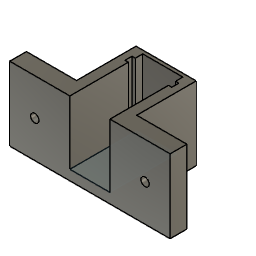
clock_light_holder (Autodesk Fusion 360 design; units mm, degrees)
Autodesk Fusion 360 part; units mm, degrees
sketch "Skizze1" plane through (0, 0, 0) normal (0, 0, 1) x (1, 0, 0)
  line L0 (0, 24) -> (16, 24)
  line L1 (16, 0) -> (0, 0)
  line L2 (2, 22) -> (14, 22)
  line L3 (0, 24) -> (-1, 24)
  line L4 (-1, 24) -> (-1, 0)
  line L5 (-1, 0) -> (0, 0)
  line L6 (16, 24) -> (17, 24)
  line L7 (17, 24) -> (17, 0)
  line L8 (17, 0) -> (16, 0)
  line L9 (2, 22) -> (1, 22)
  line L10 (1, 22) -> (1, 20)
  line L11 (1, 20) -> (2, 20)
  line L12 (15, 20) -> (15, 22)
  line L13 (15, 22) -> (14, 22)
  line L14 (15, 20) -> (2, 20)
  line L15 (2, 20) -> (2, 0)
  line L16 (14, 20) -> (14, 0)
  constraint coincident L1.end L5.end
  constraint perpendicular L3 L4
  constraint perpendicular L6 L7
  constraint perpendicular L9 L10
  constraint perpendicular L11 L12
  constraint coincident L1 L15.end
  constraint perpendicular L1 L15
  constraint coincident L14 L16.start
  constraint coincident L1 L16.end
  constraint perpendicular L1 L16
extrude "Extrusion1" add sketch "Skizze1" along normal blind 2
sketch "Skizze2" plane through (0, 0, 2) normal (0, 0, 1) x (-1, 0, 0)
  line L0 (-17, -24) -> (1, -24)
  line L1 (1, -24) -> (1, 0)
  line L2 (1, 0) -> (-17, 0)
  line L3 (-17, 0) -> (-17, -24)
  line L4 (-2, 0) -> (-2, -20)
  line L5 (-2, -20) -> (-1, -20)
  line L6 (-1, -20) -> (-1, -22)
  line L7 (-1, -22) -> (-15, -22)
  line L8 (-15, -22) -> (-15, -20)
  line L9 (-15, -20) -> (-14, -20)
  line L10 (-14, -20) -> (-14, 0)
  line L11 (-2, -20) -> (-14, -20)
  constraint coincident L2 L4.start
  constraint perpendicular L0 L4
  constraint perpendicular L4 L5
  constraint perpendicular L5 L6
  constraint perpendicular L6 L7
  constraint perpendicular L7 L8
  constraint perpendicular L8 L9
  constraint coincident L2 L10.end
  constraint perpendicular L2 L10
  constraint perpendicular L10 L11
extrude "Extrusion2" add sketch "Skizze2" along normal blind 1 contours L0 L1 L2 L3 L4 L5 L6 L7 L8 L9 L10 | L2 L4 L10 L11
sketch "Skizze3" plane through (0, 0, 3) normal (0, 0, 1) x (-1, 0, 0)
  line L0 (-15, -20) -> (-1, -20)
  line L1 (-1, -20) -> (-1, -22)
  line L2 (-1, -22) -> (-15, -22)
  line L3 (-15, -22) -> (-15, -20)
  line L4 (-17, 0) -> (-17, -24)
  line L5 (-17, -24) -> (1, -24)
  line L6 (1, -24) -> (1, 0)
  line L7 (1, 0) -> (-17, 0)
  line L8 (-2, -20) -> (-2, 0)
  line L9 (-14, -20) -> (-14, 0)
  constraint coincident L0 L8.start
  constraint coincident L7 L8.end
  constraint perpendicular L7 L8
  constraint coincident L0 L9.start
  constraint coincident L7 L9.end
  constraint perpendicular L7 L9
extrude "Extrusion3" add sketch "Skizze3" along normal blind 19 contours L0 L1 L2 L3 L4 L5 L6 L7 L8 L9
sketch "Skizze4" plane through (0, 0, 22) normal (0, 0, 1) x (-1, 0, 0)
  line L0 (-2, -20) -> (-1, -20)
  line L1 (-1, -20) -> (-1, -22)
  line L2 (-1, -22) -> (-15, -22)
  line L3 (-15, -22) -> (-15, -20)
  line L4 (-15, -20) -> (-14, -20)
  line L5 (-14, -20) -> (-14, 0)
  line L6 (-14, 0) -> (-17, 0)
  line L7 (-17, 0) -> (-17, -24)
  line L8 (-17, -24) -> (1, -24)
  line L9 (1, -24) -> (1, 0)
  line L10 (1, 0) -> (-2, 0)
  line L11 (-2, 0) -> (-2, -20)
  line L12 (-2, -22) -> (-2, -24)
  line L13 (-14, -22) -> (-14, -24)
  constraint coincident L2 L12.start
  constraint coincident L8 L12.end
  constraint perpendicular L8 L12
  constraint coincident L2 L13.start
  constraint coincident L8 L13.end
  constraint perpendicular L8 L13
extrude "Extrusion4" cut sketch "Skizze4" against normal blind 19 contours L2 L8 L12 L13
sketch "Skizze5" plane through (0, 0, 3) normal (0, 0, 1) x (-1, 0, 0)
  line L0 (-14, 0) -> (-14, -20)
  line L1 (-14, -20) -> (-2, -20)
  line L2 (-2, -20) -> (-2, 0)
  line L3 (-2, 0) -> (-14, 0)
sketch "Skizze6" plane through (0, 0, 3) normal (0, 0, 1) x (1, 0, 0)
sketch "Skizze7" plane through (0, 0, 0) normal (0, 0, 1) x (1, 0, 0)
  line L0 (-1, 0) -> (-16, 0)
  line L1 (-16, 0) -> (-16, 5)
  line L2 (-16, 5) -> (-1, 5)
  line L3 (-1, 5) -> (-1, 0)
  line L4 (17, 0) -> (17, 5)
  line L5 (17, 5) -> (32, 5)
  line L6 (32, 5) -> (32, 0)
  line L7 (32, 0) -> (17, 0)
  constraint horizontal L0
  constraint perpendicular L0 L1
  constraint perpendicular L1 L2
  constraint perpendicular L0 L3
  constraint perpendicular L0 L4
  constraint perpendicular L4 L5
  constraint perpendicular L5 L6
  constraint perpendicular L4 L7
extrude "Extrusion5" add sketch "Skizze7" along normal blind 22
hole "Bohrung1" at (24.5, 5, 11) direction (0, -1, 0) diameter 2.5 depth 5 tip angle 180 countersink diameter 4.5 countersink angle 90
hole "Bohrung2" at (-8.5, 5, 11) direction (0, -1, 0) diameter 2.5 depth 5 tip angle 180 countersink diameter 4.5 countersink angle 90
extrude "Extrusion6" cut 1 faces at (14.6667, 20, 9) along direction (0, -1, 0) blind 1
extrude "Extrusion7" add 1 faces at (1.3333, 22, 9) along direction (0, -1, 0) blind 1
sketch "Skizze8" plane through (0, 0, 3) normal (0, 0, 1) x (-1, 0, 0)
  line L0 (-14, -21) -> (-14, -24)
  line L1 (-14, -24) -> (-2, -24)
  line L2 (-2, -24) -> (-2, -21)
  line L3 (-2, -21) -> (-14, -21)
  line L4 (-2, -23) -> (-14, -23)
  line L5 (-14, -23) -> (-14, -24)
  line L6 (-14, -24) -> (-2, -24)
  line L7 (-2, -24) -> (-2, -23)
  line L8 (-2, -23) -> (-14, -23)
  line L9 (-14, -23) -> (-14, -24)
  constraint coincident L2 L4.start
  constraint coincident L0 L4.end
  constraint perpendicular L0 L4
  constraint coincident L0.end L1.start
  constraint perpendicular L1 L5
  constraint coincident L1.end L2.start
  constraint perpendicular L4 L7
  constraint perpendicular L1 L9
extrude "Extrusion8" add sketch "Skizze8" along normal blind 19 contours L0 L1 L2 L4 L5 L6 L7 L8 L9
sketch "Skizze9" plane through (0, 24, 0) normal (0, 1, 0) x (-1, 0, 0)
  line L0 (1, 22) -> (-17, 22)
  line L1 (-17, 22) -> (-17, 0)
  line L2 (-17, 0) -> (1, 0)
  line L3 (1, 0) -> (1, 22)
  line L4 (-8, 0) -> (-8, 9)
  constraint midpoint L2 L4.start
  constraint perpendicular L2 L4
hole "Bohrung3" at (8, 24, 9) direction (0, -1, 0) diameter 8 depth 9 tip angle 180
extrude "Extrusion9" cut 1 faces at (14.6667, 19, 9) along direction (0, -1, 0) blind 1.5
extrude "Extrusion10" add 1 faces at (1.3333, 21, 9) along direction (0, -1, 0) blind 1.4
extrude "Extrusion11" add 1 faces at (8, 23, 19) along direction (0, -1, 0) blind 1.2
extrude "Extrusion12" cut 1 faces at (8, 24, 19) along direction (0, -1, 0) blind 1.2
